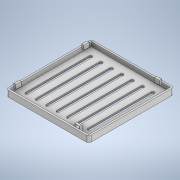
# Autodesk Inventor part: Topp
Saved by Autodesk Inventor 2021 (Build 250183000, 183)
## iProperties
Created: 2025-01-06
Part Number: Topp
Material: Generic
Document SubType Name: Sheet Metal
Designer: 22liatho
Density: 1 g/cm^3
Appearance: Default
Sheet Metal Rule: Default
Author: 22liatho
Autodesk Inventor part; units mm, degrees
ref_plane "YZ Plane" through (0, 0, 0) normal (1, 0, 0) x (0, 1, 0)
sketch "Sketch1" plane through (0, 0, 0) normal (0, 1, 0) x (-1, 0, 0)
  line L0 (0, 0) -> (-91.1, 0)
  line L1 (-91.1, 0) -> (-91.1, -94.1)
  line L2 (-91.1, -94.1) -> (0, -94.1)
  line L3 (0, -94.1) -> (0, 0)
  dimension "d0" = 91.1
  dimension "d1" = 94.1
  constraints: 8 end point, 2 parallel, 1 horizontal, 1 perpendicular
  measures "d0" distance between parallel lines of L1 L3
  measures "d1" distance between parallel lines of L2 L0
extrude "Extrusion1" add sketch "Sketch1" along normal blind 2
sketch "Sketch2" plane through (0, 2, 0) normal (0, 1, 0) x (1, 0, 0)
  line L0 (-2, -2) -> (93.1, -2)
  line L1 (93.1, -2) -> (93.1, 96.1)
  line L2 (93.1, 96.1) -> (-2, 96.1)
  line L3 (-2, 96.1) -> (-2, -2)
  line L4 (91.1, 94.1) -> (0, 94.1) projected
  line L5 (0, 0) -> (91.1, 0) projected
  line L6 (91.1, 0) -> (91.1, 94.1) projected
  line L7 (0, 94.1) -> (0, 0) projected
  line L8 (91.1, 0) -> (91.1, 94.1) projected
  line L9 (91.1, 94.1) -> (0, 94.1) projected
  line L10 (0, 94.1) -> (0, 0) projected
  line L11 (0, 0) -> (91.1, 0) projected
  line L12 (0, 0) -> (91.1, 0)
  line L13 (91.1, 0) -> (91.1, 94.1)
  line L14 (91.1, 94.1) -> (0, 94.1)
  line L15 (0, 94.1) -> (0, 0)
  dimension "d4" = 2
  dimension "d5" = 2
  dimension "d6" = 2
  dimension "d7" = 2
  constraints: 16 end point, 4 parallel, 2 horizontal, 2 perpendicular
  measures "d4" distance between parallel lines of L2 L4
  measures "d5" distance between parallel lines of L0 L5
  measures "d6" distance between parallel lines of L6 L1
  measures "d7" distance between parallel lines of L3 L7
extrude "Extrusion2" add sketch "Sketch2" along normal blind 5 and the other way blind 2
sketch "Sketch3" plane through (91.1, 2, 0) normal (0, 0, -1) x (-1, 0, 0)
  line L0 (10, 3) -> (16, 3)
  line L1 (16, 3) -> (16, 8)
  line L2 (16, 8) -> (10, 8)
  line L3 (10, 8) -> (10, 3)
  line L4 (0, 0) -> (0, 5) projected
  line L5 (0, 5) -> (91.1, 5) projected
  point P0 (91.1, -2)
  dimension "d12" = 10
  dimension "d13" = 2
  dimension "d14" = 3
  dimension "d15" = 6
  constraints: 8 end point, 2 parallel, 1 horizontal, 1 perpendicular
  measures "d12" distance between parallel lines of L4 L3
  measures "d13" distance between parallel lines of L5 L0
  measures "d14" distance between parallel lines of L2 L5
  measures "d15" distance between parallel lines of L1 L3
extrude "Extrusion3" add sketch "Sketch3" along normal blind 2.5
sketch "Sketch4" plane through (91.1, 2, 0) normal (0, 0, 1) x (1, 0, 0)
  line L0 (-14.55, 6.8) -> (-11.45, 6.8)
  line L1 (-11.45, 6.8) -> (-11.45, 6.2)
  line L2 (-11.45, 6.2) -> (-14.55, 6.2)
  line L3 (-14.55, 6.2) -> (-14.55, 6.8)
  line L4 (-10, 8) -> (-10, 5) projected
  line L5 (-16, 5) -> (-16, 8) projected
  line L6 (-16, 8) -> (-10, 8) projected
  line L7 (-93.1, 5) -> (2, 5) projected
  point P0 (-91.1, -2)
  dimension "d18" = 3.1
  dimension "d19" = 0.6
  dimension "d20" = 1.45
  dimension "d21" = 1.45
  dimension "d22" = 1.2
  dimension "d23" = 1.2
  constraints: 8 end point, 2 parallel, 1 horizontal, 1 perpendicular
  measures "d18" distance of L0.start L0.end
  measures "d19" distance of L0.end L1.end
  measures "d20" distance between parallel lines of L4 L1
  measures "d21" distance between parallel lines of L5 L3
  measures "d22" distance between parallel lines of L6 L0
  measures "d23" distance between parallel lines of L7 L2
extrude "Extrusion4" cut sketch "Sketch4" against normal blind 2 contours L0 L1 L2 L3
chamfer "Chamfer1" distance 1 distance2 1.6 1 edges at (78.1, 8.8, 0) measured on face at (78.6167, 9.6, 0)
chamfer "Chamfer2" distance 1 distance2 1.6 1 edges at (76.55, 8.5, 0) measured on face at (78.6167, 7.4, 0)
chamfer "Chamfer3" distance 1 distance2 1.6 1 edges at (78.1, 8.2, 0) measured on face at (78.6167, 7.4, 0)
chamfer "Chamfer4" distance 1 distance2 1.6 1 edges at (79.65, 8.5, 0) measured on face at (80.6167, 8.6, 0)
sketch "Sketch5" plane through (0, 2, 0) normal (1, 0, 0) x (0, 0, -1)
  line L0 (5, 3) -> (11, 3)
  line L1 (11, 3) -> (11, 8)
  line L2 (11, 8) -> (5, 8)
  line L3 (5, 8) -> (5, 3)
  line L4 (96.1, 5) -> (-2, 5) projected
  line L5 (0, 5) -> (0, 0) projected
  point P0 (0, -2)
  dimension "d38" = 3
  dimension "d39" = 6
  dimension "d40" = 2
  dimension "d41" = 5
  constraints: 8 end point, 2 parallel, 1 horizontal, 1 perpendicular
  measures "d38" distance between parallel lines of L4 L2
  measures "d39" distance between parallel lines of L3 L1
  measures "d40" distance between parallel lines of L4 L0
  measures "d41" distance between parallel lines of L5 L3
extrude "Extrusion5" add sketch "Sketch5" along normal blind 2.5
sketch "Sketch6" plane through (0, 2, 0) normal (-1, 0, 0) x (0, 0, 1)
  line L0 (-9.55, 6.8) -> (-6.45, 6.8)
  line L1 (-6.45, 6.8) -> (-6.45, 6.2)
  line L2 (-6.45, 6.2) -> (-9.55, 6.2)
  line L3 (-9.55, 6.2) -> (-9.55, 6.8)
  line L4 (-11, 8) -> (-5, 8) projected
  line L5 (-5, 8) -> (-5, 5) projected
  point P0 (0, -2)
  point P1 (-8, 6.8)
  point P2 (-8, 8)
  point P3 (-5, 6.5)
  point P4 (-6.45, 6.5)
  dimension "d44" = 0.6
  dimension "d45" = 3.1
  constraints: 8 end point, 4 midpoint, 2 parallel, 1 horizontal, 1 horizontal alignment, 1 perpendicular, 1 vertical alignment
  measures "d44" distance of L0.end L1.end
  measures "d45" distance of L0.start L0.end
extrude "Extrusion6" cut sketch "Sketch6" against normal blind 2
chamfer "Chamfer5" distance 1 distance2 1.6 1 edges at (0, 8.8, -8) measured on face at (0, 9.6, -7.4833)
chamfer "Chamfer6" distance 1 distance2 1.6 1 edges at (0, 8.2, -8) measured on face at (0, 7.4, -7.4833)
chamfer "Chamfer7" distance 1 distance2 1.6 1 edges at (0, 8.5, -9.55) measured on face at (0, 8.6, -5.4833)
chamfer "Chamfer8" distance 1 distance2 1.6 1 edges at (0, 8.5, -6.45) measured on face at (0, 8.6, -5.4833)
ref_plane "Work Plane2" through (-2, 7, -47.05) normal (0, 0, 1) x (1, 0, 0)
ref_plane "Work Plane1" through (-2, 7, -29.05) normal (0, 0, 1) x (1, 0, 0)
mirror "Mirror1" about plane through (-2, 7, -47.05) normal (0, 0, 1) of "Extrusion5", "Extrusion6", "Chamfer5", "Chamfer8", "Chamfer7", "Chamfer6"
mirror "Mirror2" about plane through (-2, 7, -47.05) normal (0, 0, 1) of "Extrusion3", "Extrusion4", "Chamfer1", "Chamfer2", "Chamfer3", "Chamfer4"
sketch "Sketch7" plane through (0, 0, 0) normal (0, -1, 0) x (1, 0, 0)
  line L0 (8, -10.5) -> (8, -83.6)
  arc A0 (8, -83.6) -> (11.5, -83.6) centre (9.75, -83.6) ccw
  line L1 (11.5, -83.6) -> (11.5, -10.5)
  arc A1 (11.5, -10.5) -> (8, -10.5) centre (9.75, -10.5) ccw
  line L2 (93.1, 2) -> (-2, 2) projected
  line L3 (-2, -96.1) -> (93.1, -96.1) projected
  line L4 (-2, 2) -> (-2, -96.1) projected
  line L5 (23.4333, -83.6) -> (23.4333, -10.5)
  arc A2 (19.9333, -83.6) -> (23.4333, -83.6) centre (21.6833, -83.6) ccw
  line L6 (19.9333, -10.5) -> (19.9333, -83.6)
  arc A3 (23.4333, -10.5) -> (19.9333, -10.5) centre (21.6833, -10.5) ccw
  line L7 (35.3667, -83.6) -> (35.3667, -10.5)
  arc A4 (31.8667, -83.6) -> (35.3667, -83.6) centre (33.6167, -83.6) ccw
  line L8 (31.8667, -10.5) -> (31.8667, -83.6)
  arc A5 (35.3667, -10.5) -> (31.8667, -10.5) centre (33.6167, -10.5) ccw
  line L9 (47.3, -83.6) -> (47.3, -10.5)
  arc A6 (43.8, -83.6) -> (47.3, -83.6) centre (45.55, -83.6) ccw
  line L10 (43.8, -10.5) -> (43.8, -83.6)
  arc A7 (47.3, -10.5) -> (43.8, -10.5) centre (45.55, -10.5) ccw
  line L11 (59.2333, -83.6) -> (59.2333, -10.5)
  arc A8 (55.7333, -83.6) -> (59.2333, -83.6) centre (57.4833, -83.6) ccw
  line L12 (55.7333, -10.5) -> (55.7333, -83.6)
  arc A9 (59.2333, -10.5) -> (55.7333, -10.5) centre (57.4833, -10.5) ccw
  line L13 (71.1667, -83.6) -> (71.1667, -10.5)
  arc A10 (67.6667, -83.6) -> (71.1667, -83.6) centre (69.4167, -83.6) ccw
  line L14 (67.6667, -10.5) -> (67.6667, -83.6)
  arc A11 (71.1667, -10.5) -> (67.6667, -10.5) centre (69.4167, -10.5) ccw
  line L15 (83.1, -83.6) -> (83.1, -10.5)
  arc A12 (79.6, -83.6) -> (83.1, -83.6) centre (81.35, -83.6) ccw
  line L16 (79.6, -10.5) -> (79.6, -83.6)
  arc A13 (83.1, -10.5) -> (79.6, -10.5) centre (81.35, -10.5) ccw
  line L17 (93.1, -96.1) -> (93.1, 2) projected
  point P0 (0, 0)
  dimension "d61" = 3.5
  dimension "d62" = 12.5
  dimension "d63" = 12.5
  dimension "d64" = 10
  dimension "d67" = 11.9333
  dimension "d72" = 10
  constraints: 28 end point, 28 point on circle, 14 centre point, 4 tangent, 2 vertical, 1 horizontal, 60 other
  measures "d61" distance between parallel lines of L1 L0
  measures "d62" distance from line of L2 A1.centre
  measures "d63" distance from line of L3 A0.centre
  measures "d64" distance between parallel lines of L4 L0
  measures "d67" distance of L1.start L5.start
  measures "d72" distance between parallel lines of L17 L15
extrude "Extrusion7" cut sketch "Sketch7" against normal through all contours A1 L1 A0 L0 | A2 L6 A3 L5 | A4 L8 A5 L7 | A6 L10 A7 L9 | A8 L12 A9 L11 | A10 L14 A11 L13 | A12 L16 A13 L15
fillet "Fillet1" radius 3 4 edges at (93.1, 3.5, 2) (-2, 3.5, 2) (93.1, 3.5, -96.1) (-2, 3.5, -96.1)
sketch "Sketch9" plane through (0, 0, 0) normal (0, -1, 0) x (1, 0, 0)
  line L0 (12.2167, -62.05) -> (12.2167, -32.05) construction
  line L1 (12.2167, -32.05) -> (19.2167, -32.05) construction
  line L2 (19.2167, -32.05) -> (19.2167, -62.05) construction
  line L3 (19.2167, -62.05) -> (12.2167, -62.05) construction
  line L4 (90.1, 2) -> (1, 2) projected
  line L5 (1, -96.1) -> (90.1, -96.1) projected
  line L6 (11.5, -10.5) -> (11.5, -83.6) projected
  line L7 (19.9333, -83.6) -> (19.9333, -10.5) projected
  spline S0 degree 2 poles (14.6875, -55.0058) (15.0116, -55.0058) (15.5951, -55.2368) (15.7977, -55.4434) knots 0 0 0 1 2 2 2
  spline S1 degree 2 poles (15.7977, -55.4434) (16.053, -55.7028) (16.3163, -56.4037) (16.3163, -56.9386) knots 0 0 0 1 2 2 2
  line L8 (16.3163, -56.9386) -> (16.3163, -57.5018)
  line L9 (16.3163, -57.5018) -> (18.1802, -57.5018)
  line L10 (18.1802, -57.5018) -> (18.1802, -58.1663)
  line L11 (18.1802, -58.1663) -> (13.1802, -58.1663)
  line L12 (13.1802, -58.1663) -> (13.1802, -56.9102)
  spline S2 degree 2 poles (13.1802, -56.9102) (13.1802, -56.4645) (13.3261, -55.8405) (13.4922, -55.6015) knots 0 0 0 1 2 2 2
  spline S3 degree 2 poles (13.4922, -55.6015) (13.6826, -55.3219) (14.2702, -55.0058) (14.6875, -55.0058) knots 0 0 0 1 2 2 2
  spline S4 degree 2 poles (14.7078, -55.6987) (14.4484, -55.6987) (14.0676, -55.877) (13.946, -56.0593) knots 0 0 0 1 2 2 2
  spline S5 degree 2 poles (13.946, -56.0593) (13.8407, -56.2173) (13.7556, -56.6387) (13.7556, -56.9507) knots 0 0 0 1 2 2 2
  line L13 (13.7556, -56.9507) -> (13.7556, -57.5018)
  line L14 (13.7556, -57.5018) -> (15.7491, -57.5018)
  line L15 (15.7491, -57.5018) -> (15.7491, -57.048)
  spline S6 degree 2 poles (15.7491, -57.048) (15.7491, -56.6428) (15.6194, -56.1444) (15.4492, -55.9823) knots 0 0 0 1 2 2 2
  spline S7 degree 2 poles (15.4492, -55.9823) (15.2993, -55.8324) (14.9468, -55.6987) (14.7078, -55.6987) knots 0 0 0 1 2 2 2
  line L16 (18.1802, -53.7781) -> (18.1802, -54.4102)
  line L17 (18.1802, -54.4102) -> (14.4282, -54.4102)
  line L18 (14.4282, -54.4102) -> (14.4282, -53.7781)
  line L19 (14.4282, -53.7781) -> (18.1802, -53.7781)
  line L20 (13.8042, -53.7335) -> (13.8042, -54.4507)
  line L21 (13.8042, -54.4507) -> (13.1478, -54.4507)
  line L22 (13.1478, -54.4507) -> (13.1478, -53.7335)
  line L23 (13.1478, -53.7335) -> (13.8042, -53.7335)
  line L24 (13.1802, -49.1752) -> (18.1802, -50.8972)
  line L25 (18.1802, -50.8972) -> (18.1802, -51.6144)
  line L26 (18.1802, -51.6144) -> (13.1802, -53.3365)
  line L27 (13.1802, -53.3365) -> (13.1802, -52.6233)
  line L28 (13.1802, -52.6233) -> (17.3334, -51.2376)
  line L29 (17.3334, -51.2376) -> (13.1802, -49.8519)
  line L30 (13.1802, -49.8519) -> (13.1802, -49.1752)
  line L31 (18.1802, -48.1015) -> (18.1802, -48.7335)
  line L32 (18.1802, -48.7335) -> (14.4282, -48.7335)
  line L33 (14.4282, -48.7335) -> (14.4282, -48.1015)
  line L34 (14.4282, -48.1015) -> (18.1802, -48.1015)
  line L35 (13.8042, -48.0569) -> (13.8042, -48.7741)
  line L36 (13.8042, -48.7741) -> (13.1478, -48.7741)
  line L37 (13.1478, -48.7741) -> (13.1478, -48.0569)
  line L38 (13.1478, -48.0569) -> (13.8042, -48.0569)
  spline S8 degree 2 poles (18.2693, -46.1606) (18.2693, -46.5374) (18.0667, -47.1898) (17.9533, -47.4045) knots 0 0 0 1 2 2 2
  line L39 (17.9533, -47.4045) -> (17.2442, -47.4045)
  line L40 (17.2442, -47.4045) -> (17.2442, -47.3721)
  spline S9 degree 2 poles (17.2442, -47.3721) (17.309, -47.2911) (17.463, -47.0723) (17.5481, -46.89) knots 0 0 0 1 2 2 2
  spline S10 degree 2 poles (17.5481, -46.89) (17.6251, -46.7319) (17.7385, -46.3429) (17.7385, -46.1363) knots 0 0 0 1 2 2 2
  spline S11 degree 2 poles (17.7385, -46.1363) (17.7385, -45.9864) (17.6697, -45.642) (17.6129, -45.5609) knots 0 0 0 1 2 2 2
  spline S12 degree 2 poles (17.6129, -45.5609) (17.536, -45.4434) (17.3617, -45.3381) (17.1834, -45.3381) knots 0 0 0 1 2 2 2
  spline S13 degree 2 poles (17.1834, -45.3381) (16.9606, -45.3381) (16.7296, -45.5812) (16.6526, -45.8932) knots 0 0 0 1 2 2 2
  spline S14 degree 2 poles (16.6526, -45.8932) (16.6243, -46.0147) (16.5432, -46.4037) (16.4987, -46.5699) knots 0 0 0 1 2 2 2
  spline S15 degree 2 poles (16.4987, -46.5699) (16.3731, -46.9994) (15.8544, -47.3883) (15.4857, -47.3883) knots 0 0 0 1 2 2 2
  spline S16 degree 2 poles (15.4857, -47.3883) (14.9752, -47.3883) (14.339, -46.6225) (14.339, -45.9904) knots 0 0 0 1 2 2 2
  spline S17 degree 2 poles (14.339, -45.9904) (14.339, -45.6784) (14.493, -45.0464) (14.6105, -44.8316) knots 0 0 0 1 2 2 2
  line L41 (14.6105, -44.8316) -> (15.2872, -44.8316)
  line L42 (15.2872, -44.8316) -> (15.2872, -44.864)
  spline S18 degree 2 poles (15.2872, -44.864) (15.0927, -45.1071) (14.8698, -45.6987) (14.8698, -46.0026) knots 0 0 0 1 2 2 2
  spline S19 degree 2 poles (14.8698, -46.0026) (14.8698, -46.3146) (15.1332, -46.7441) (15.3966, -46.7441) knots 0 0 0 1 2 2 2
  spline S20 degree 2 poles (15.3966, -46.7441) (15.6356, -46.7441) (15.8666, -46.4888) (15.9395, -46.2052) knots 0 0 0 1 2 2 2
  spline S21 degree 2 poles (15.9395, -46.2052) (15.976, -46.0674) (16.0489, -45.719) (16.0935, -45.5285) knots 0 0 0 1 2 2 2
  spline S22 degree 2 poles (16.0935, -45.5285) (16.1988, -45.1152) (16.681, -44.6938) (17.0984, -44.6938) knots 0 0 0 1 2 2 2
  spline S23 degree 2 poles (17.0984, -44.6938) (17.3415, -44.6938) (17.771, -44.8843) (17.929, -45.0707) knots 0 0 0 1 2 2 2
  spline S24 degree 2 poles (17.929, -45.0707) (18.0951, -45.2692) (18.2693, -45.7757) (18.2693, -46.1606) knots 0 0 0 1 2 2 2
  line L43 (18.1802, -43.4621) -> (18.1802, -44.0942)
  line L44 (18.1802, -44.0942) -> (14.4282, -44.0942)
  line L45 (14.4282, -44.0942) -> (14.4282, -43.4621)
  line L46 (14.4282, -43.4621) -> (18.1802, -43.4621)
  line L47 (13.8042, -43.4175) -> (13.8042, -44.1347)
  line L48 (13.8042, -44.1347) -> (13.1478, -44.1347)
  line L49 (13.1478, -44.1347) -> (13.1478, -43.4175)
  line L50 (13.1478, -43.4175) -> (13.8042, -43.4175)
  spline S25 degree 2 poles (16.3042, -39.4507) (17.2523, -39.4507) (18.2855, -40.3624) (18.2855, -41.1241) knots 0 0 0 1 2 2 2
  spline S26 degree 2 poles (18.2855, -41.1241) (18.2855, -41.9062) (17.2199, -42.8016) (16.3042, -42.8016) knots 0 0 0 1 2 2 2
  spline S27 degree 2 poles (16.3042, -42.8016) (15.3642, -42.8016) (14.3228, -41.8778) (14.3228, -41.1241) knots 0 0 0 1 2 2 2
  spline S28 degree 2 poles (14.3228, -41.1241) (14.3228, -40.3624) (15.3601, -39.4507) (16.3042, -39.4507) knots 0 0 0 1 2 2 2
  spline S29 degree 2 poles (16.3042, -40.1031) (15.5749, -40.1031) (14.8658, -40.6339) (14.8658, -41.1241) knots 0 0 0 1 2 2 2
  spline S30 degree 2 poles (14.8658, -41.1241) (14.8658, -41.6144) (15.5749, -42.1493) (16.3042, -42.1493) knots 0 0 0 1 2 2 2
  spline S31 degree 2 poles (16.3042, -42.1493) (17.0133, -42.1493) (17.7426, -41.6144) (17.7426, -41.1241) knots 0 0 0 1 2 2 2
  spline S32 degree 2 poles (17.7426, -41.1241) (17.7426, -40.6379) (17.0254, -40.1031) (16.3042, -40.1031) knots 0 0 0 1 2 2 2
  line L51 (18.1802, -35.8567) -> (18.1802, -36.4888)
  line L52 (18.1802, -36.4888) -> (16.0408, -36.4888)
  spline S33 degree 2 poles (16.0408, -36.4888) (15.7815, -36.4888) (15.3358, -36.5374) (15.2021, -36.6104) knots 0 0 0 1 2 2 2
  spline S34 degree 2 poles (15.2021, -36.6104) (15.0603, -36.6874) (14.9225, -36.9629) (14.9225, -37.1979) knots 0 0 0 1 2 2 2
  spline S35 degree 2 poles (14.9225, -37.1979) (14.9225, -37.4329) (15.1737, -37.9313) (15.3763, -38.1703) knots 0 0 0 1 2 2 2
  line L53 (15.3763, -38.1703) -> (18.1802, -38.1703)
  line L54 (18.1802, -38.1703) -> (18.1802, -38.8024)
  line L55 (18.1802, -38.8024) -> (14.4282, -38.8024)
  line L56 (14.4282, -38.8024) -> (14.4282, -38.1703)
  line L57 (14.4282, -38.1703) -> (14.8455, -38.1703)
  spline S36 degree 2 poles (14.8455, -38.1703) (14.5902, -37.8867) (14.3228, -37.3397) (14.3228, -37.0318) knots 0 0 0 1 2 2 2
  spline S37 degree 2 poles (14.3228, -37.0318) (14.3228, -36.4807) (15.0522, -35.8567) (15.745, -35.8567) knots 0 0 0 1 2 2 2
  line L58 (15.745, -35.8567) -> (18.1802, -35.8567)
  point P0 (0, 0)
  dimension "d81" = 30
  dimension "d82" = 34.05
  dimension "d83" = 34.05
  dimension "d84" = 0.7167
  dimension "d85" = 7
  dimension "d86" = 0.7167
  constraints: 1 vertical, 2 other
  measures "d81" distance of L0.start L0.end
  measures "d82" distance between parallel lines of L4 L1
  measures "d83" distance between parallel lines of L5 L3
  measures "d84" distance between parallel lines of L6 L0
  measures "d85" distance between parallel lines of L0 L2
  measures "d86" distance between parallel lines of L7 L2
extrude "Extrusion9" cut sketch "Sketch9" against normal blind 1
equation "\"d20\" = d21"
equation "\"d22\" = d23"
equation "\"GapSize\" = Thickness"
equation "\"BendRadius\" = Thickness"
equation "\"MinimumRemnant\" = 2 * Thickness"
equation "\"BendReliefDepth\" = 0.5 * Thickness"
equation "\"BendReliefWidth\" = Thickness"
equation "\"CornerReliefSize\" = 4 * Thickness"
equation "\"JacobiRadiusSize\" = Thickness"
equation "\"TransitionRadius\" = BendRadius"
equation "\"d82\" = d83"
equation "\"d84\" = d86"
equation "\"Thickness\" = 0.5"
body "Solid1"
